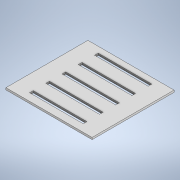
# Autodesk Inventor part: end_part_ferrite
Saved by Autodesk Inventor 2020 (Build 240168000, 168)
## iProperties
Created: 2021-01-27
Part Number: end_part_ferrite
Material: Generic
Document SubType Name: Modeling
Designer: apat475
Density: 1 g/cm^3
Appearance: Default
Author: apat475
Autodesk Inventor part; units mm, degrees
ref_plane "YZ Plane" through (0, 0, 0) normal (1, 0, 0) x (0, 1, 0)
ref_plane "XZ Plane" through (0, 0, 0) normal (0, 1, 0) x (-1, 0, 0)
ref_plane "XY Plane" through (0, 0, 0) normal (0, 0, 1) x (1, 0, 0)
sketch "Sketch1" plane through (0, 0, 0) normal (0, 1, 0) x (-1, 0, 0)
  line L0 (93.9879, 146.0349) -> (-256.0121, 146.0349)
  line L1 (-256.0121, 146.0349) -> (-256.0121, -186.9651)
  line L2 (-256.0121, -186.9651) -> (93.9879, -186.9651)
  line L3 (93.9879, -186.9651) -> (93.9879, 146.0349)
  line L4 (27.9879, 116.0349) -> (-190.0121, 116.0349)
  line L5 (-190.0121, 116.0349) -> (-190.0121, 101.0349)
  line L6 (-190.0121, 101.0349) -> (27.9879, 101.0349)
  line L7 (27.9879, 101.0349) -> (27.9879, 116.0349)
  line L8 (27.9879, 50.0349) -> (-190.0121, 50.0349)
  line L9 (-190.0121, 50.0349) -> (-190.0121, 35.0349)
  line L10 (-190.0121, 35.0349) -> (27.9879, 35.0349)
  line L11 (27.9879, 35.0349) -> (27.9879, 50.0349)
  line L12 (27.9879, -15.9651) -> (-190.0121, -15.9651)
  line L13 (-190.0121, -15.9651) -> (-190.0121, -30.9651)
  line L14 (-190.0121, -30.9651) -> (27.9879, -30.9651)
  line L15 (27.9879, -30.9651) -> (27.9879, -15.9651)
  line L16 (27.9879, -81.9651) -> (-190.0121, -81.9651)
  line L17 (-190.0121, -81.9651) -> (-190.0121, -96.9651)
  line L18 (-190.0121, -96.9651) -> (27.9879, -96.9651)
  line L19 (27.9879, -96.9651) -> (27.9879, -81.9651)
  line L20 (27.9879, -147.9651) -> (-190.0121, -147.9651)
  line L21 (-190.0121, -147.9651) -> (-190.0121, -162.9651)
  line L22 (-190.0121, -162.9651) -> (27.9879, -162.9651)
  line L23 (27.9879, -162.9651) -> (27.9879, -147.9651)
  point P0 (0, 0)
  dimension "d0" = 333
  dimension "d1" = 350
  dimension "d2" = 66
  dimension "d6" = 51
  dimension "d7" = 51
  dimension "d8" = 51
  dimension "d9" = 15
  dimension "d10" = 15
  dimension "d11" = 15
  dimension "d12" = 15
  dimension "d13" = 30
  dimension "d16" = 51
  dimension "d17" = 15
  constraints: 48 end point, 12 parallel, 6 horizontal, 6 perpendicular, 6 point on line
  measures "d0" distance of L2.end L0.start
  measures "d1" distance of L1.end L2.end
  measures "d2" distance between parallel lines of L3 L19
  measures "d6" distance between parallel lines of L16 L14
  measures "d7" distance between parallel lines of L10 L12
  measures "d8" distance between parallel lines of L6 L8
  measures "d9" distance of L14.end L12.start
  measures "d10" distance of L10.end L8.start
  measures "d11" distance of L6.end L4.start
  measures "d12" distance of L18.end L16.start
  measures "d13" distance between parallel lines of L0 L4
  measures "d16" distance between parallel lines of L20 L18
  measures "d17" distance of L22.end L20.start
extrude "Extrusion2" add sketch "Sketch1" against normal blind 8
body "Solid2"
